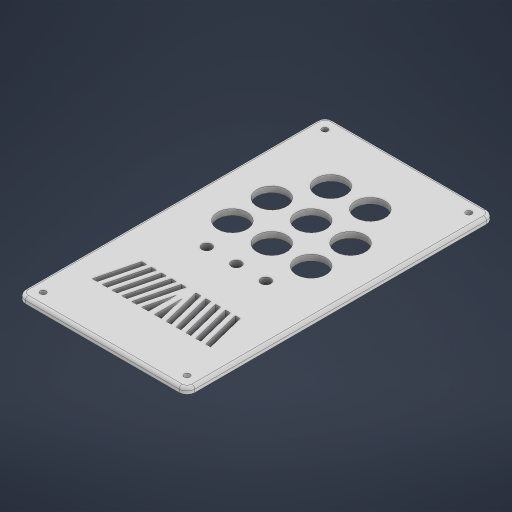
# Autodesk Inventor part: TUTUP CASING
Saved by Autodesk Inventor 2024 (Build 280153000, 153)
## iProperties
Created: 2025-06-23
Part Number: TUTUP CASING
Material: Generic
Document SubType Name: Modeling
Designer: ASUS
Density: 1 g/cm^3
Appearance: Default
Author: ASUS
Autodesk Inventor part; units mm, degrees
ref_plane "YZ Plane" through (0, 0, 0) normal (1, 0, 0) x (0, 1, 0)
ref_plane "XZ Plane" through (0, 0, 0) normal (0, 1, 0) x (-1, 0, 0)
ref_plane "XY Plane" through (0, 0, 0) normal (0, 0, 1) x (1, 0, 0)
sketch "Sketch2" plane through (0, 0, 0) normal (0, 1, 0) x (-1, 0, 0)
  line L0 (-39, 86) -> (39, 86)
  arc A0 (43, 82) -> (39, 86) centre (39, 82) ccw
  line L1 (43, 82) -> (43, -66)
  arc A1 (39, -70) -> (43, -66) centre (39, -66) ccw
  line L2 (39, -70) -> (-39, -70)
  arc A2 (-43, -66) -> (-39, -70) centre (-39, -66) ccw
  line L3 (-43, -66) -> (-43, 82)
  arc A3 (-39, 86) -> (-43, 82) centre (-39, 82) ccw
  circle A4 centre (0, -20) radius 7.5
  circle A5 centre (-20, -20) radius 7.5
  circle A6 centre (20, -20) radius 7.5
  circle A7 centre (0, 0) radius 7.5
  circle A8 centre (-20, 0) radius 7.5
  circle A9 centre (20, 0) radius 7.5
  circle A10 centre (-10, -40) radius 7.5
  circle A11 centre (10, -40) radius 7.5
  circle A12 centre (-36.5, 79.5) radius 1.5
  circle A13 centre (36.5, 79.5) radius 1.5
  circle A14 centre (-36.5, -63.5) radius 1.5
  circle A15 centre (36.5, -63.5) radius 1.5
  line L4 (-30, 61) -> (-27.5, 61)
  line L5 (-30, 61) -> (-25, 41)
  line L6 (-25, 61) -> (-20, 41)
  line L7 (-20, 61) -> (-15, 41)
  line L8 (-15, 61) -> (-10, 41)
  line L9 (-10, 61) -> (-5, 41)
  line L10 (-5, 61) -> (-1.5, 47)
  line L11 (30, 61) -> (25, 41)
  line L12 (25, 61) -> (20, 41)
  line L13 (20, 61) -> (15, 41)
  line L14 (15, 61) -> (10, 41)
  line L15 (10, 61) -> (5, 41)
  line L16 (5, 61) -> (1.5, 47)
  line L17 (-20, 61) -> (-17.5, 61)
  line L18 (-22.5, 41) -> (-25, 41)
  line L19 (-10, 61) -> (-7.5, 61)
  line L20 (-12.5, 41) -> (-15, 41)
  line L21 (25, 41) -> (22.5, 41)
  line L22 (27.5, 61) -> (30, 61)
  line L23 (15, 41) -> (12.5, 41)
  line L24 (17.5, 61) -> (20, 61)
  line L25 (7.5, 61) -> (10, 61)
  line L26 (22.5, 41) -> (27.5, 61)
  line L27 (20, 41) -> (17.5, 41)
  line L28 (25, 61) -> (22.5, 61)
  line L29 (17.5, 41) -> (22.5, 61)
  line L30 (12.5, 41) -> (17.5, 61)
  line L31 (15, 61) -> (12.5, 61)
  line L32 (10, 41) -> (7.5, 41)
  line L33 (7.5, 41) -> (12.5, 61)
  line L34 (-22.5, 41) -> (-27.5, 61)
  line L35 (-12.5, 41) -> (-17.5, 61)
  line L36 (-22.5, 61) -> (-25, 61)
  line L37 (-17.5, 41) -> (-20, 41)
  line L38 (-17.5, 41) -> (-22.5, 61)
  line L39 (-7.5, 41) -> (-10, 41)
  line L40 (-12.5, 61) -> (-15, 61)
  line L41 (-7.5, 41) -> (-12.5, 61)
  line L42 (2.5, 41) -> (7.5, 61)
  line L43 (-2.5, 41) -> (-7.5, 61)
  line L44 (5, 41) -> (2.5, 41)
  line L45 (-2.5, 41) -> (-5, 41)
  line L46 (5, 61) -> (1.5, 61)
  line L47 (1.5, 61) -> (1.5, 47)
  line L48 (-5, 61) -> (-1.5, 61)
  line L49 (-1.5, 61) -> (-1.5, 47)
  circle A16 centre (15, 18) radius 2.5
  circle A17 centre (0, 18) radius 2.5
  circle A18 centre (-15, 18) radius 2.5
  point P0 (-43, -66)
  point P1 (39, -70)
  point P2 (43, 82)
  dimension "d6" = 3.5
  dimension "d7" = 3.5
  dimension "d8" = 90
  dimension "d10" = 5
  dimension "d11" = 5
  dimension "d12" = 5
  constraints: 100 end point, 19 centre point, 8 point on circle, 6 equal length, 4 horizontal, 1 perpendicular
  measures "d6" distance of L16.start L46.end
  measures "d7" distance of L10.start L48.end
  measures "d8" angle of L48 L49
  measures "d10" diameter of A16
  measures "d11" diameter of A17
  measures "d12" diameter of A18
extrude "Extrusion2" add sketch "Sketch2" along normal blind 3
fillet "Fillet2" radius 1.5 8 edges at (41.8284, 3, -68.8284) (0, 3, -70) (-41.8284, 3, -68.8284) (-43, 3, 8) (-41.8284, 3, 84.8284) (0, 3, 86) (41.8284, 3, 84.8284) (43, 3, 8)
body "Solid2"
